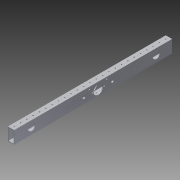
# Autodesk Inventor part: chassis side rail
Saved by Autodesk Inventor 2014 SP1 (Build 180222100, 222)
## iProperties
Created: 2014-01-04
Part Number: chassis side rail
Material: Aluminum 6061
Document SubType Name: Modeling
Designer: Arpan
Density: 2.71 g/cm^3
Appearance: Aluminum - Flat
Mass: 580.286 g
Surface Area: 1734.53 cm^2
Volume: 214.128 cm^3
Author: Arpan
Autodesk Inventor part; units mm, degrees
ref_plane "YZ Plane" through (0, 0, 0) normal (1, 0, 0) x (0, 1, 0)
ref_plane "XZ Plane" through (0, 0, 0) normal (0, 1, 0) x (-1, 0, 0)
ref_plane "XY Plane" through (0, 0, 0) normal (0, 0, 1) x (1, 0, 0)
sketch "Sketch1" plane through (0, 0, 0) normal (0, 0, 1) x (1, 0, 0)
  line L0 (0, 0) -> (-25.4, 0)
  line L1 (-25.4, 0) -> (-25.4, 50.8)
  line L2 (-25.4, 50.8) -> (0, 50.8)
  line L3 (0, 50.8) -> (0, 0)
  line L4 (-2.54, 48.26) -> (-22.86, 48.26)
  line L5 (-22.86, 48.26) -> (-22.86, 2.54)
  line L6 (-22.86, 2.54) -> (-2.54, 2.54)
  line L7 (-2.54, 2.54) -> (-2.54, 48.26)
  line L8 (-25.4, 50.8) -> (-12.7, 50.8)
  line L9 (-12.7, 50.8) -> (-12.7, 50.7238)
  line L10 (-12.7, 50.7238) -> (-12.7762, 50.8)
  line L11 (-12.7, 50.7238) -> (-12.6238, 50.8)
  dimension "d0" = 25.4
  dimension "d1" = 50.8
  dimension "d2" = 2.54
  dimension "d32" = 12.7
  dimension "d33" = 0.0762
  dimension "d34" = 135
  dimension "d35" = 135
  constraints: 24 end point, 4 parallel, 3 perpendicular, 2 point on line, 1 horizontal, 1 midpoint, 3 other
  measures "d0" distance of L1.end L2.end
  measures "d1" distance of L2.end L0.start
  measures "d2" distance between parallel lines of L2 L4
  measures "d32" distance of L1.end L8.end
  measures "d33" distance of L8.end L9.end
  measures "d34" angle of L2 L10
  measures "d35" angle of L2 L11
extrude "Extrusion1" add sketch "Sketch1" along normal blind 685.8
sketch "Sketch2" plane through (0, 0, 0) normal (1, 0, 0) x (0, 0, -1)
  line L0 (0, 50.8) -> (0, 0) projected
  line L1 (-685.8, 0) -> (-685.8, 50.8) projected
  line L2 (0, 0) -> (-685.8, 0) projected
  line L3 (-685.8, 0) -> (-685.8, 25.4)
  line L4 (-685.8, 25.4) -> (-660.4, 25.4)
  line L5 (-660.4, 25.4) -> (-660.4, 0)
  line L6 (0, 25.4) -> (-25.4, 25.4)
  line L7 (-25.4, 25.4) -> (-25.4, 0)
  dimension "d5" = 25.4
  dimension "d6" = 25.4
  dimension "d7" = 25.4
  constraints: 10 end point, 4 perpendicular, 2 midpoint, 2 point on line
  measures "d5" distance of L1.start L3.end
  measures "d6" distance of L3.end L4.end
  measures "d7" distance of L6.start L6.end
extrude "Extrusion2" cut sketch "Sketch2" against normal blind 685.8
sketch "Sketch3" plane through (-25.4, 50.8, 0) normal (-1, 0, 0) x (0, 0, 1)
  line L0 (25.4, -50.8) -> (88.9, -50.8)
  line L1 (88.9, -50.8) -> (88.9, -23.8125)
  circle A0 centre (88.9, -23.8125) radius 14.2875
  circle A1 centre (590.55, -23.8125) radius 14.2875
  line L2 (88.9, -50.8) -> (322.58, -50.8)
  line L3 (322.58, -50.8) -> (322.58, -23.8125)
  line L4 (322.58, -23.8125) -> (322.58, -26.9875)
  circle A2 centre (322.58, -26.9875) radius 19.05
  line L5 (0, -25.4) -> (25.4, -25.4) projected
  line L6 (685.8, 0) -> (685.8, -25.4) projected
  line L7 (0, -25.4) -> (0, 0) projected
  line L8 (660.4, -50.8) -> (590.55, -50.8)
  line L9 (590.55, -50.8) -> (590.55, -23.8125)
  point P0 (0, -50.8)
  dimension "d11" = 26.9875
  dimension "d12" = 28.575
  dimension "d14" = 28.575
  dimension "d16" = 3.175
  dimension "d18" = 38.1
  dimension "d68" = 233.68
  dimension "d70" = 267.97
  dimension "d71" = 63.5
  dimension "d72" = 69.85
  dimension "d73" = 1.5875
  dimension "d74" = 1.5875
  constraints: 14 end point, 4 perpendicular, 3 centre point, 2 coincident, 1 parallel, 1 point on line
  measures "d11" distance of L0.end L1.end
  measures "d12" diameter of A0
  measures "d14" diameter of A1
  measures "d16" distance of L3.end L4.end
  measures "d18" diameter of A2
  measures "d68" horizontal distance of L4.end L1.end
  measures "d70" horizontal distance of L9.end L4.end
  measures "d71" distance of L0.start L0.end
  measures "d72" distance of L8.start L8.end
  measures "d73" distance from line of L9.end L5
  measures "d74" distance from line of L3.end L5
extrude "Extrusion3" cut sketch "Sketch3" against normal blind 685.8
sketch "Sketch4" plane through (-25.4, 50.8, 0) normal (-1, 0, 0) x (0, 0, 1)
  circle A0 centre (322.58, -26.9875) radius 19.05 projected
  line L0 (0, -25.4) -> (0, 0) projected
  line L1 (322.58, -26.9875) -> (298.7548, -26.9875)
  circle A1 centre (298.7548, -26.9875) radius 2.54
  line L2 (322.58, -26.9875) -> (346.4052, -26.9875)
  circle A2 centre (346.4052, -26.9875) radius 2.54
  line L3 (322.58, -26.9875) -> (265.43, -26.9875)
  line L4 (322.58, -26.9875) -> (379.73, -26.9875)
  circle A3 centre (265.43, -26.9875) radius 5.08
  circle A4 centre (379.73, -26.9875) radius 5.08
  point P0 (0, -50.8)
  dimension "d21" = 23.8252
  dimension "d22" = 5.08
  dimension "d23" = 23.8252
  dimension "d24" = 5.08
  dimension "d25" = 57.15
  dimension "d26" = 57.15
  dimension "d27" = 10.16
  constraints: 8 end point, 4 centre point, 4 coincident, 3 collinear, 1 perpendicular
  measures "d21" distance of L1.start L1.end
  measures "d22" diameter of A1
  measures "d23" distance of L1.start L2.end
  measures "d24" diameter of A2
  measures "d25" distance of L1.start L3.end
  measures "d26" distance of L1.start L4.end
  measures "d27" diameter of A3
extrude "Extrusion4" cut sketch "Sketch4" against normal blind 25.4 contours A1 L3 L1 | L1 L3 A1 | A2 L4 L2 | L2 L4 A2 | A3 | A4
sketch "Sketch5" plane through (-25.4, 50.8, 0) normal (-1, 0, 0) x (0, 0, 1)
  arc A0 (357.2379, -7.8193) -> (357.0276, -12.0844) centre (355.8548, -9.8888) ccw projected
  arc A1 (357.0276, -12.0844) -> (357.2379, -7.8193) centre (358.4107, -10.0149) ccw projected
  arc A2 (288.8902, -10.4426) -> (288.8855, -6.1723) centre (290.1673, -8.3061) ccw projected
  arc A3 (288.8855, -6.1723) -> (288.8902, -10.4426) centre (287.6083, -8.3089) ccw projected
  circle A4 centre (287.6083, -8.3089) radius 2.4892
  circle A5 centre (358.4107, -10.0149) radius 2.4892
  point P0 (0, -50.8)
  constraints: 2 coincident, 6 other
extrude "Extrusion5" cut sketch "Sketch5" against normal blind 25.4 contours A1 A5 | A3 A4
sketch "Sketch6" plane through (0, 0, 685.8) normal (0, 0, 1) x (1, 0, 0)
  line L0 (-25.4, 25.4) -> (-22.86, 25.4) projected
  line L1 (-2.54, 25.4) -> (0, 25.4) projected
  line L2 (0, 25.4) -> (0, 50.8) projected
  line L3 (0, 50.8) -> (-25.4, 50.8) projected
  line L4 (-25.4, 50.8) -> (-25.4, 25.4) projected
  line L5 (-12.7, 50.8) -> (-12.7, 50.7238)
  line L6 (-12.7, 50.7238) -> (-12.7762, 50.8)
  line L7 (-12.7, 50.7238) -> (-12.6238, 50.8)
  line L8 (-25.4, 50.8) -> (-25.4, 38.1)
  line L9 (-25.4, 38.1) -> (-25.4, 25.4)
  line L10 (0, 50.8) -> (0, 38.1)
  line L11 (-25.4, 38.1) -> (-25.3238, 38.1)
  line L12 (0, 38.1) -> (-0.0762, 38.1)
  line L13 (-0.0762, 38.1) -> (0, 38.1762)
  line L14 (-0.0762, 38.1) -> (0, 38.0238)
  line L15 (-25.3238, 38.1) -> (-25.4, 38.1762)
  line L16 (-25.3238, 38.1) -> (-25.4, 38.0238)
  line L17 (-25.4, 25.4) -> (-25.3238, 25.4)
  line L18 (-25.3238, 25.4) -> (-25.4, 25.4762)
  line L19 (0, 25.4) -> (-0.0762, 25.4)
  line L20 (-0.0762, 25.4) -> (0, 25.4762)
  point P0 (0, 0)
  dimension "d36" = 0.0762
  dimension "d37" = 135
  dimension "d38" = 135
  dimension "d39" = 12.7
  dimension "d40" = 0.0762
  dimension "d41" = 0.0762
  dimension "d42" = 0.0762
  dimension "d43" = 0.0762
  constraints: 32 end point, 10 point on line, 5 perpendicular, 3 midpoint, 3 parallel, 2 collinear
  measures "d36" distance of L5.start L5.end
  measures "d37" angle of L6 L3
  measures "d38" angle of L3 L7
  measures "d39" distance of L3.end L8.end
  measures "d40" distance of L8.end L11.end
  measures "d41" distance of L10.end L12.end
  measures "d42" distance of L0.start L17.end
  measures "d43" distance of L1.end L19.end
extrude "Extrusion6" cut sketch "Sketch6" against normal blind 685.8
sketch "Sketch7" plane through (-25.4, 0, 660.4) normal (0, 0, 1) x (1, 0, 0)
  line L0 (0.0762, 25.4) -> (0, 25.4) projected
  line L1 (0, 0) -> (0, 25.4) projected
  line L2 (25.4, 0) -> (0, 0) projected
  line L3 (25.4, 25.4) -> (25.4, 0) projected
  line L4 (25.4, 25.4) -> (25.3238, 25.4) projected
  line L5 (25.3238, 25.4) -> (25.4, 25.3238)
  line L6 (0.0762, 25.4) -> (0, 25.3238)
  line L7 (0, 0) -> (0, 12.7)
  line L8 (0, 12.7) -> (0.0762, 12.7)
  line L9 (0.0762, 12.7) -> (0, 12.7762)
  line L10 (0.0762, 12.7) -> (0, 12.6238)
  line L11 (25.4, 0) -> (25.4, 12.7)
  line L12 (25.4, 12.7) -> (25.3238, 12.7)
  line L13 (25.3238, 12.7) -> (25.4, 12.6238)
  line L14 (25.3238, 12.7) -> (25.4, 12.7762)
  line L15 (12.7, 0) -> (12.7, 0.0762)
  line L16 (12.7, 0.0762) -> (12.6238, 0)
  line L17 (12.7, 0.0762) -> (12.7762, 0)
  dimension "d46" = 135
  dimension "d47" = 135
  dimension "d48" = 12.7
  dimension "d50" = 0.0762
  dimension "d51" = 0.0762
  constraints: 26 end point, 8 perpendicular, 8 point on line, 3 midpoint, 1 collinear
  measures "d46" angle of L3 L5
  measures "d47" angle of L1 L6
  measures "d48" distance of L1.start L7.end
  measures "d50" distance of L11.end L12.end
  measures "d51" distance of L15.start L15.end
extrude "Extrusion7" cut sketch "Sketch7" against normal blind 685.8
sketch "Sketch8" plane through (0, 50.8, 685.8) normal (0, 1, 0) x (1, 0, 0)
  line L0 (-12.6238, 685.8) -> (-12.6238, 0) projected
  line L1 (-12.6238, 685.8) -> (0, 685.8) projected
  line L2 (-12.6238, 685.8) -> (-12.7, 685.8)
  line L3 (-12.7, 685.8) -> (-12.7, 673.1)
  circle A0 centre (-12.7, 673.1) radius 2.0828
  dimension "d54" = 0.0762
  dimension "d55" = 12.7
  dimension "d56" = 4.1656
  constraints: 4 end point, 1 centre point, 1 coincident, 1 collinear, 1 parallel
  measures "d54" distance of L0.start L2.end
  measures "d55" distance of L2.end L3.end
  measures "d56" diameter of A0
extrude "Extrusion8" cut sketch "Sketch8" against normal blind 685.8 contours A0 L0 | L0 A0
pattern_linear "Rectangular Pattern1" count 27 spacing 25.4 along (0, 0, 1) of "Extrusion8"
sketch "Sketch9" plane through (0, 50.8, 685.8) normal (1, 0, 0) x (0, 0, -1)
  line L0 (0, 0) -> (25.4, 0)
  line L1 (25.4, 0) -> (25.4, -25.4)
  line L2 (25.4, -25.4) -> (0, -25.4)
  line L3 (0, -25.4) -> (0, 0)
  line L4 (685.8, 0) -> (660.4, 0)
  line L5 (660.4, 0) -> (660.4, -25.4)
  line L6 (660.4, -25.4) -> (685.8, -25.4)
  line L7 (685.8, -25.4) -> (685.8, 0)
  point P0 (685.8, -50.8)
  dimension "d62" = 25.4
  dimension "d63" = 25.4
  dimension "d64" = 25.4
  dimension "d65" = 25.4
  constraints: 16 end point, 4 parallel, 2 horizontal, 2 perpendicular
  measures "d62" distance of L1.end L2.end
  measures "d63" distance of L0.end L1.end
  measures "d64" distance of L6.end L5.end
  measures "d65" distance of L6.end L4.start
extrude "Extrusion9" cut sketch "Sketch9" against normal blind 25.4
body "Solid1"
